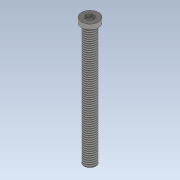
# Autodesk Inventor part: perno_simple
Saved by Autodesk Inventor 2022 (Build 260153000, 153)
## iProperties
Created: 2022-03-21
Part Number: perno_simple
Material: Generic
Document SubType Name: Sheet Metal
Designer: ferna
Density: 1 g/cm^3
Sheet Metal Rule: Default_mm
Appearance: Galvanized
Author: ferna
Autodesk Inventor part; units mm, degrees
ref_plane "YZ Plane" through (0, 0, 0) normal (1, 0, 0) x (0, 1, 0)
ref_plane "XZ Plane" through (0, 0, 0) normal (0, 1, 0) x (-1, 0, 0)
ref_plane "XY Plane" through (0, 0, 0) normal (0, 0, 1) x (1, 0, 0)
sketch "Sketch1" plane through (0, 0, 0) normal (0, 1, 0) x (-1, 0, 0)
  circle A0 centre (0, 0) radius 2.45
  dimension "d0" = 4.9
  constraints: 1 centre point, 1 coincident
  measures "d0" diameter of A0
extrude "Extrusion1" add sketch "Sketch1" along normal blind 50
sketch "Sketch2" plane through (0, 50, 0) normal (0, 1, 0) x (1, 0, 0)
  circle A0 centre (0, 0) radius 3.5
  dimension "d3" = 7
  constraints: 1 centre point, 1 coincident
  measures "d3" diameter of A0
extrude "Extrusion2" add sketch "Sketch2" along normal blind 2
thread "Thread1" size "M5x0.8" class "6g" standard "ANSI Metric M Profile" full length
sketch "Sketch3" plane through (0, 52, 0) normal (0, 1, 0) x (1, 0, 0)
  line L0 (0.866, 1.5) -> (1.7321, 0)
  line L1 (1.7321, 0) -> (0.866, -1.5)
  line L2 (0.866, -1.5) -> (-0.866, -1.5)
  line L3 (-0.866, -1.5) -> (-1.7321, 0)
  line L4 (-1.7321, 0) -> (-0.866, 1.5)
  line L5 (-0.866, 1.5) -> (0.866, 1.5)
  point P0 (0, 0)
  point P1 (0, 0)
  dimension "d8" = 3
  constraints: 12 end point, 1 coincident, 13 other
  measures "d8" distance between parallel lines of L2 L5
extrude "Extrusion3" cut sketch "Sketch3" against normal blind 1
equation "\"BendRadius\" = Thickness"
equation "\"BendReliefWidth\" = Thickness"
equation "\"BendReliefDepth\" = 0.5 * Thickness"
equation "\"CornerReliefSize\" = 4 * Thickness"
equation "\"MinimumRemnant\" = 2 * Thickness"
equation "\"TransitionRadius\" = BendRadius"
equation "\"JacobiRadiusSize\" = BendRadius"
equation "\"GapSize\" = Thickness"
equation "\"Thickness\" = 0.5"
body "Solid1"
